Autodesk Inventor part; units mm, degrees
(part 2 of 2)
sketch "Sketch21" plane through (6.35, 0, 0) normal (1, 0, 0) x (0, 0, -1)
  circle A0 centre (-38.2612, -63.5431) radius 1.9939 projected
  circle A1 centre (-38.2612, -63.5431) radius 1.9939
  circle A2 centre (43.0188, -63.5431) radius 1.9939 projected
  circle A3 centre (43.0188, -63.5431) radius 1.9939
  line L0 (-35.2132, -58.3752) -> (-35.2132, -68.7109)
  line L1 (-42.0712, -70.6551) -> (-42.0712, -56.4311)
  line L2 (-36.9448, -55.5472) -> (-40.101, -53.9363)
  line L3 (-41.462, -52.597) -> (-42.0712, -51.4492)
  line L4 (-36.9448, -71.5389) -> (-40.101, -73.1498)
  line L5 (-41.462, -74.4891) -> (-42.0712, -75.6369)
  arc A4 (-41.462, -52.597) -> (-40.101, -53.9363) centre (-38.6576, -51.1084) ccw
  arc A5 (-40.101, -73.1498) -> (-41.462, -74.4891) centre (-38.6576, -75.9777) ccw
  arc A6 (-36.9448, -71.5389) -> (-35.2132, -68.7109) centre (-38.3882, -68.7109) ccw
  arc A7 (-35.2132, -58.3752) -> (-36.9448, -55.5472) centre (-38.3882, -58.3752) ccw
  line L6 (46.8288, -56.4311) -> (46.8288, -70.6551)
  line L7 (39.9708, -68.7109) -> (39.9708, -58.3752)
  line L8 (41.7024, -55.5472) -> (44.852, -53.9397)
  line L9 (46.213, -52.6004) -> (46.8288, -51.4403)
  line L10 (41.7024, -71.5389) -> (44.852, -73.1465)
  line L11 (46.213, -74.4858) -> (46.8288, -75.6459)
  arc A8 (46.213, -74.4858) -> (44.852, -73.1465) centre (43.4086, -75.9744) ccw
  arc A9 (39.9708, -68.7109) -> (41.7024, -71.5389) centre (43.1458, -68.7109) ccw
  arc A10 (44.852, -53.9397) -> (46.213, -52.6004) centre (43.4086, -51.1117) ccw
  arc A11 (41.7024, -55.5472) -> (39.9708, -58.3752) centre (43.1458, -58.3752) ccw
  line L12 (46.8288, -51.4403) -> (46.8288, -75.6459)
  line L13 (-42.0712, -51.4492) -> (-42.0712, -75.6369)
  point P0 (0, 0)
  point P1 (-37.8414, -63.5431)
  point P2 (-37.853, -70.6551)
  point P3 (-37.853, -56.4311)
  point P4 (-40.9926, -53.4812)
  point P5 (-40.9926, -73.6049)
  point P6 (43.3998, -70.6551)
  point P7 (45.7436, -53.4846)
  dimension "d135" = 14.224
  dimension "d149" = 3.9878
  dimension "d168" = 145
  dimension "d169" = 145
  dimension "d170" = 117.04
  dimension "d171" = 117.04
  dimension "d172" = 2.032
  dimension "d173" = 2.032
  dimension "d175" = 3.175
  dimension "d176" = 3.1561
  dimension "d177" = 3.1561
  dimension "d179" = 7.112
  dimension "d181" = 145
  dimension "d182" = 145
  dimension "d183" = 117.04
  dimension "d184" = 117.04
  dimension "d185" = 3.175
  dimension "d187" = 3.175
  dimension "d188" = 3.1496
  dimension "d189" = 2.0443
  dimension "d190" = 3.1496
  constraints: 28 end point, 16 point on circle, 16 tangent, 10 centre point, 6 equal radius, 6 point on line, 2 coincident, 2 parallel, 2 vertical
  measures "d135" distance of point (-37.853, -70.655) point (-37.853, -56.431)
  measures "d149" diameter of A0
  measures "d168" angle of L2 L3
  measures "d169" angle of L5 L4
  measures "d170" angle of L4 L0
  measures "d171" angle of L0 L2
  measures "d172" vertical distance of point (-40.993, -53.481) L3.end
  measures "d173" vertical distance of point (-40.993, -73.605) L5.end
  measures "d175" radius of A4
  measures "d176" horizontal distance of L2.start L2.end
  measures "d177" horizontal distance of L4.start L4.end
  measures "d179" vertical distance of point (43.4, -70.655) A3.centre
  measures "d181" angle of L8 L9
  measures "d182" angle of L11 L10
  measures "d183" angle of L10 L7
  measures "d184" angle of L7 L8
  measures "d185" radius of A8
  measures "d187" radius of A10
  measures "d188" horizontal distance of L8.start L8.end
  measures "d189" vertical distance of L9.end point (45.744, -53.485)
  measures "d190" horizontal distance of L10.start L10.end
extrude "Extrusion13" add sketch "Sketch21" along normal blind 8.89
fillet "Fillet6" radius 0.508 11 edges at (16.002, 50.7569, -21.4288) (11.684, 50.7569, -2.3788) (16.002, 50.7569, 16.6712) (18.161, -43.0961, 48.4212) (16.002, -47.0966, 48.4212) (18.161, -51.0971, 48.4212) (19.7104, -216.9591, 3.2854) (18.2245, -216.9591, 2.2854) (17.3482, -216.9591, -1.7184) (18.2245, -216.9591, -5.7222) (19.7104, -216.9591, -6.7222)
body "Solid1"
